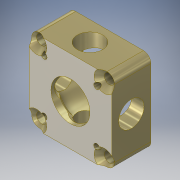
# Autodesk Inventor part: Pump_Adapter
Saved by Autodesk Inventor 2016 (Build 200138000, 138)
## iProperties
Created: 2015-06-30
Part Number: Pump_Adapter
Material: Generic
Document SubType Name: Modeling
Designer: bastli
Density: 1 g/cm^3
Appearance: Gold - Metal
Mass: 11.2099 g
Surface Area: 57.0387 cm^2
Volume: 11.2099 cm^3
Author: bastli
Autodesk Inventor part; units mm, degrees
ref_plane "YZ Plane" through (0, 0, 0) normal (1, 0, 0) x (0, 1, 0)
ref_plane "XZ Plane" through (0, 0, 0) normal (0, 1, 0) x (-1, 0, 0)
ref_plane "XY Plane" through (0, 0, 0) normal (0, 0, 1) x (1, 0, 0)
sketch "Sketch1" plane through (0, 0, 0) normal (0, 0, 1) x (1, 0, 0)
  circle A0 centre (-20, 20) radius 1.5 construction
  circle A1 centre (-20, 20) radius 4.5 construction
  circle A2 centre (20, 20) radius 1.5 construction
  circle A3 centre (20, 20) radius 4.5 construction
  circle A4 centre (20, -20) radius 1.5 construction
  circle A5 centre (20, -20) radius 4.5 construction
  circle A6 centre (-20, -20) radius 1.5 construction
  circle A7 centre (-20, -20) radius 4.5 construction
  arc A8 (25, 20) -> (20, 25) centre (20, 20) ccw construction
  line L0 (-20, 25) -> (20, 25) construction
  arc A9 (-20, 25) -> (-25, 20) centre (-20, 20) ccw construction
  line L1 (-25, -20) -> (-25, 20) construction
  arc A10 (-25, -20) -> (-20, -25) centre (-20, -20) ccw construction
  line L2 (20, -25) -> (-20, -25) construction
  arc A11 (20, -25) -> (25, -20) centre (20, -20) ccw construction
  line L3 (25, 20) -> (25, -20) construction
  circle A12 centre (20, -20) radius 4.5 construction
  circle A13 centre (-20, -20) radius 4.5 construction
  circle A14 centre (-20, 20) radius 4.5 construction
  circle A15 centre (20, 20) radius 4.5 construction
  circle A16 centre (0, 0) radius 10.5 construction
  arc A17 (24.4, 20) -> (20, 24.4) centre (20, 20) ccw
  line L4 (24.4, 20) -> (24.4, -20)
  arc A18 (20, -24.4) -> (24.4, -20) centre (20, -20) ccw
  line L5 (20, -24.4) -> (-20, -24.4)
  arc A19 (-24.4, -20) -> (-20, -24.4) centre (-20, -20) ccw
  line L6 (-24.4, -20) -> (-24.4, 20)
  arc A20 (-20, 24.4) -> (-24.4, 20) centre (-20, 20) ccw
  line L7 (-20, 24.4) -> (20, 24.4)
  point P0 (0, 0)
  dimension "d0" = 0.6
  constraints: 8 end point, 8 point on circle, 4 centre point, 4 coincident, 7 other
  measures "d0" distance between parallel lines of L0 L7
extrude "Extrusion1" add sketch "Sketch1" along normal blind 23.1
sketch "Sketch2" plane through (0, 0, 23.1) normal (0, 0, 1) x (1, 0, 0)
  point P0 (0, 0)
  point P1 (20, 20)
  point P2 (20, -20)
  point P3 (-20, -20)
  point P4 (-20, 20)
hole "Hole1" at (20, 20, 23.1) at (20, -20, 23.1) at (-20, -20, 23.1) at (-20, 20, 23.1) direction (0, 0, -1) diameter 3.4 end up to face face through (-6.6667, 8.1333, 0) facing (0, 0, -1)
sketch "Sketch3" plane through (0, 0, 23.1) normal (0, 0, 1) x (1, 0, 0)
  line L0 (-15.5, 15.5) -> (15.5, 15.5) construction
  line L1 (15.5, 15.5) -> (15.5, -15.5) construction
  line L2 (15.5, -15.5) -> (-15.5, -15.5) construction
  line L3 (-15.5, -15.5) -> (-15.5, 15.5) construction
  line L4 (-15.5, 15.5) -> (15.5, -15.5) construction
  line L5 (15.5, 15.5) -> (-15.5, -15.5) construction
  point P0 (0, 0)
  dimension "d10" = 31
  dimension "d11" = 31
  constraints: 12 end point, 4 coincident, 2 midpoint, 2 parallel, 1 horizontal, 1 perpendicular
  measures "d10" distance of L1.end L2.end
  measures "d11" distance of L0.end L1.end
hole "Hole2" at (15.5, 15.5, 23.1) at (15.5, -15.5, 23.1) at (-15.5, -15.5, 23.1) at (-15.5, 15.5, 23.1) direction (0, 0, -1) diameter 3.4 end up to face face through (6.2425, -6.2909, 0) facing (0, 0, -1)
sketch "Sketch5" plane through (0, 0, 23.1) normal (0, 0, 1) x (1, 0, 0)
  circle A0 centre (0, 0) radius 11.5
  dimension "d22" = 23
  constraints: 1 centre point, 1 coincident
  measures "d22" diameter of A0
extrude "Extrusion3" cut sketch "Sketch5" against normal up to surface (23.1 mm away)
sketch "Sketch6" plane through (0, 0, 23.1) normal (0, 0, 1) x (1, 0, 0)
  circle A0 centre (20, -20) radius 1.7 projected
  circle A1 centre (20, -20) radius 3
  circle A2 centre (20, 20) radius 1.7 projected
  circle A3 centre (20, 20) radius 3
  circle A4 centre (-20, -20) radius 1.7 projected
  circle A5 centre (-20, -20) radius 3
  circle A6 centre (-20, 20) radius 3
  point P0 (0, 0)
  dimension "d25" = 6
  dimension "d26" = 6
  dimension "d28" = 6
  dimension "d29" = 6
  constraints: 4 centre point, 4 coincident
  measures "d25" diameter of A1
  measures "d26" diameter of A3
  measures "d28" diameter of A5
  measures "d29" diameter of A6
extrude "Extrusion4" cut sketch "Sketch6" against normal blind 15.7
sketch "Sketch7" plane through (0, 0, 0) normal (0, 0, -1) x (-1, 0, 0)
  circle A0 centre (-15.5, -15.5) radius 1.7 projected
  circle A1 centre (-15.5, 15.5) radius 1.7 projected
  circle A2 centre (15.5, 15.5) radius 1.7 projected
  circle A3 centre (15.5, -15.5) radius 1.7 projected
  circle A4 centre (-15.5, -15.5) radius 3
  circle A5 centre (-15.5, 15.5) radius 3
  circle A6 centre (15.5, -15.5) radius 3
  circle A7 centre (15.5, 15.5) radius 3
  point P0 (0, 0)
  dimension "d32" = 6
  dimension "d33" = 6
  dimension "d34" = 6
  dimension "d35" = 6
  constraints: 4 centre point
  measures "d32" diameter of A4
  measures "d33" diameter of A5
  measures "d34" diameter of A7
  measures "d35" diameter of A6
extrude "Extrusion5" cut sketch "Sketch7" against normal blind 15.7
chamfer "Chamfer3" distance 3 angle 45 4 edges at (-23, 20, 23.1) (-23, -20, 23.1) (17, -20, 23.1) (17, 20, 23.1)
chamfer "Chamfer1" distance 1.2 angle 45 8 edges at (20, -18.3, 7.4) (20, 21.7, 7.4) (-20, 21.7, 7.4) (-20, -18.3, 7.4) (-15.5, 17.2, 15.7) (-15.5, -13.8, 15.7) (15.5, -13.8, 15.7) (15.5, 17.2, 15.7)
derived "Honlite Axes Adapter.ipt"
sketch "Sketch8" plane through (-24.4, -20, 0) normal (-1, 0, 0) x (0, 0, 1)
  line L0 (0, 0) -> (0, 40) projected
  line L1 (0, 0) -> (21.5, 0) projected
  line L2 (23.1, 35.9208) -> (23.1, 4.0792) projected
  line L3 (0, 40) -> (21.5, 40) projected
  line L4 (0, 40) -> (23.1, 40) construction
  line L5 (0, 0) -> (0, 40) construction
  line L6 (23.1, 40) -> (0, 0) construction
  line L7 (0, 0) -> (23.1, 0) construction
  line L8 (0, 0) -> (23.1, 0) construction
  line L9 (23.1, 3) -> (23.1, -3) construction
  line L10 (23.1, 0) -> (0, 40) construction
  circle A0 centre (11.55, 20) radius 7.5
  point P0 (0, 20)
  dimension "d42" = 15
  constraints: 6 end point, 1 centre point, 1 midpoint, 1 perpendicular, 2 other
  measures "d42" diameter of A0
extrude "Extrusion6" cut sketch "Sketch8" against normal up to surface round surface about axis through (0, 0, 23.1) along (0, 0, -1) radius 11.5 far side no
pattern_circular "Circular Pattern1" count 4 over 360 about axis through (0, 0, 23.1) along (0, 0, -1) of "Extrusion6"
derived "Pump_Head.ipt"
sketch "Sketch9" plane through (0, 0, 0) normal (0, 0, -1) x (-1, 0, 0)
  circle A0 centre (0, 0) radius 16.9203
  circle A1 centre (-15.5, -15.5) radius 3 projected
  dimension "d49" = 2
  constraints: 1 centre point, 1 coincident
extrude "Extrusion7" cut sketch "Sketch9" against normal blind 17.1 contours A0
chamfer "Chamfer2" distance 2 angle 45 12 edges at (-8.1317, -8.1317, 17.1) (-11.1282, -2.9005, 18.4664) (-11.127, 2.9052, 18.4645) (-8.1317, 8.1317, 17.1) (-2.9005, 11.1282, 18.4664) (2.9052, 11.127, 18.4645) (8.1317, 8.1317, 17.1) (11.1282, 2.9005, 18.4664) (11.127, -2.9052, 18.4645) (8.1317, -8.1317, 17.1) (2.9005, -11.1282, 18.4664) (-2.9052, -11.127, 18.4645)
body "Solid1"
